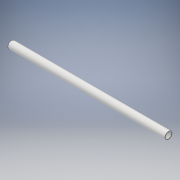
# Autodesk Inventor part: Ground_Tracker_CrossTube
Saved by Autodesk Inventor 2018 (Build 220112000, 112)
## iProperties
Created: 2018-09-27
Part Number: Ground_Tracker_CrossTube
Material: PVC-Piping
Document SubType Name: Modeling
Designer: Bradley
Density: 1.4 g/cm^3
Appearance: Smooth - White
Mass: 527.61 g
Surface Area: 1666.03 cm^2
Volume: 376.864 cm^3
Author: Bradley
Autodesk Inventor part; units mm, degrees
ref_plane "YZ Plane" through (0, 0, 0) normal (1, 0, 0) x (0, 1, 0)
ref_plane "XZ Plane" through (0, 0, 0) normal (0, 1, 0) x (-1, 0, 0)
ref_plane "XY Plane" through (0, 0, 0) normal (0, 0, 1) x (1, 0, 0)
sketch "Sketch1" plane through (0, 0, 0) normal (1, 0, 0) x (0, 1, 0)
  circle A0 centre (0, 0) radius 21.082
  circle A1 centre (0, 0) radius 17.526
  dimension "d0" = 42.164
  dimension "d1" = 35.052
  constraints: 2 centre point, 2 coincident
  measures "d0" diameter of A0
  measures "d1" diameter of A1
extrude "Extrusion1" add sketch "Sketch1" along normal mid plane 914.4
body "Solid1"
